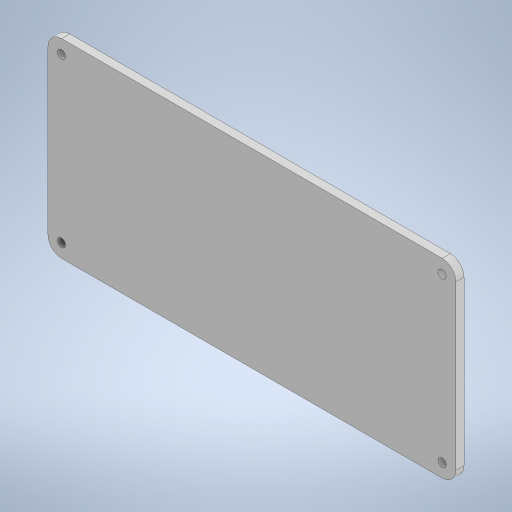
# Autodesk Inventor part: Charger ShroudPlate - EthanMockup
Saved by Autodesk Inventor 2023 (Build 270158000, 158)
## iProperties
Created: 2023-01-17
Part Number: Charger ShroudPlate - EthanMockup
Material: Generic
Document SubType Name: Modeling
Designer: ethan
Density: 1 g/cm^3
Appearance: Default
Author: ethan
Autodesk Inventor part; units mm, degrees
ref_plane "YZ Plane" through (0, 0, 0) normal (1, 0, 0) x (0, 1, 0)
ref_plane "XZ Plane" through (0, 0, 0) normal (0, 1, 0) x (-1, 0, 0)
ref_plane "XY Plane" through (0, 0, 0) normal (0, 0, 1) x (1, 0, 0)
sketch "Sketch1" plane through (0, 0, 0) normal (0, 0, 1) x (1, 0, 0)
  line L0 (0, 0) -> (150, 0)
  line L1 (150, 0) -> (150, 70)
  line L2 (150, 70) -> (0, 70)
  line L3 (0, 70) -> (0, 0)
  line L4 (5, 65) -> (145, 65) construction
  line L5 (145, 65) -> (145, 5) construction
  line L6 (145, 5) -> (5, 5) construction
  line L7 (5, 5) -> (5, 65) construction
  circle A0 centre (5, 65) radius 1.5
  circle A1 centre (5, 5) radius 1.5
  circle A2 centre (145, 5) radius 1.5
  circle A3 centre (145, 65) radius 1.5
  dimension "d0" = 150
  dimension "d1" = 70
  dimension "d2" = 5
  dimension "d3" = 5
  dimension "d4" = 60
  dimension "d5" = 140
  dimension "d6" = 3
  dimension "d7" = 3
  dimension "d8" = 3
  dimension "d9" = 3
  constraints: 16 end point, 4 centre point, 4 coincident, 4 parallel, 2 horizontal, 2 perpendicular
  measures "d0" distance of L2.end L1.end
  measures "d1" distance of L1.end L0.end
  measures "d2" distance between parallel lines of L2 L4
  measures "d3" distance between parallel lines of L3 L7
  measures "d4" distance of L4.end L5.end
  measures "d5" distance of L4.start L4.end
  measures "d6" diameter of A0
  measures "d7" diameter of A1
  measures "d8" diameter of A2
  measures "d9" diameter of A3
extrude "Extrusion1" add sketch "Sketch1" along normal blind 3
fillet "Fillet1" radius 5 4 edges at (0, 70, 1.5) (0, 0, 1.5) (150, 0, 1.5) (150, 70, 1.5)
body "Solid1"
